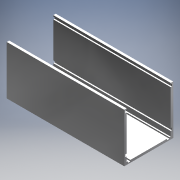
# Autodesk Inventor part: CompactSlidePart1
Saved by Autodesk Inventor 2019 (Build 230136000, 136)
## iProperties
Created: 2017-11-11
Part Number: CompactSlidePart1
Material: Aluminum 6061
Document SubType Name: Modeling
Designer: User
Density: 2.7 g/cm^3
Appearance: Aluminum - Flat
Mass: 1825.11 g
Surface Area: 2444.35 cm^2
Volume: 675.966 cm^3
Author: User
Autodesk Inventor part; units mm, degrees
ref_plane "YZ Plane" through (0, 0, 0) normal (1, 0, 0) x (0, 1, 0)
ref_plane "XZ Plane" through (0, 0, 0) normal (0, 1, 0) x (-1, 0, 0)
ref_plane "XY Plane" through (0, 0, 0) normal (0, 0, 1) x (1, 0, 0)
sketch "Sketch1" plane through (0, 0, 0) normal (1, 0, 0) x (0, 1, 0)
  line L0 (0, 0) -> (-127, 0)
  line L1 (-127, 0) -> (-127, -127)
  line L2 (-127, -127) -> (0, -127)
  line L3 (0, -127) -> (0, -120.65)
  line L4 (0, -6.35) -> (0, 0)
  line L5 (0, -6.35) -> (-3.175, -6.35)
  line L6 (-3.175, -6.35) -> (-3.175, -3.175)
  line L7 (-3.175, -3.175) -> (-9.525, -3.175)
  line L8 (-9.525, -3.175) -> (-9.525, -6.35)
  line L9 (-3.175, -6.35) -> (0, -6.35)
  line L10 (0, -120.65) -> (-3.175, -120.65)
  line L11 (-3.175, -120.65) -> (-3.175, -123.825)
  line L12 (-3.175, -123.825) -> (-9.525, -123.825)
  line L13 (-9.525, -123.825) -> (-9.525, -120.65)
  line L14 (0, -120.65) -> (-3.175, -120.65)
  line L15 (-120.65, -6.35) -> (-120.65, -9.525)
  line L16 (-120.65, -9.525) -> (-123.825, -9.525)
  line L17 (-123.825, -9.525) -> (-123.825, -15.875)
  line L18 (-123.825, -15.875) -> (-120.65, -15.875)
  line L19 (-120.65, -9.525) -> (-120.65, -6.35)
  line L20 (-120.65, -120.65) -> (-120.65, -117.475)
  line L21 (-120.65, -117.475) -> (-123.825, -117.475)
  line L22 (-123.825, -117.475) -> (-123.825, -111.125)
  line L23 (-123.825, -111.125) -> (-120.65, -111.125)
  line L24 (-120.65, -120.65) -> (-120.65, -117.475)
  line L25 (-120.65, -111.125) -> (-120.65, -15.875)
  line L26 (-120.65, -6.35) -> (-107.95, -6.35)
  line L27 (-107.95, -6.35) -> (-107.95, -3.175)
  line L28 (-107.95, -3.175) -> (-101.6, -3.175)
  line L29 (-101.6, -3.175) -> (-101.6, -6.35)
  line L30 (-120.65, -6.35) -> (-107.95, -6.35)
  line L31 (-101.6, -6.35) -> (-9.525, -6.35)
  line L32 (-120.65, -120.65) -> (-107.95, -120.65)
  line L33 (-107.95, -120.65) -> (-107.95, -123.825)
  line L34 (-107.95, -123.825) -> (-101.6, -123.825)
  line L35 (-101.6, -123.825) -> (-101.6, -120.65)
  line L36 (-9.525, -120.65) -> (-101.6, -120.65)
  line L37 (-107.95, -120.65) -> (-120.65, -120.65)
  dimension "d0" = 127
  dimension "d1" = 127
  dimension "d2" = 6.35
  dimension "d3" = 120.65
  dimension "d4" = 114.3
  dimension "d5" = 3.175
  dimension "d9" = 3.175
  dimension "d10" = 3.175
  dimension "d11" = 3.175
  dimension "d12" = 6.35
  dimension "d13" = 3.175
  dimension "d14" = 3.175
  dimension "d15" = 6.35
  dimension "d16" = 3.175
  dimension "d17" = 3.175
  dimension "d18" = 6.35
  dimension "d21" = 12.7
  dimension "d22" = 3.175
  dimension "d23" = 6.35
  dimension "d24" = 12.7
  dimension "d25" = 3.175
  dimension "d26" = 6.35
  constraints: 76 end point, 46 perpendicular, 4 horizontal, 3 parallel
  measures "d0" distance of L0.start L0.end
  measures "d1" distance of L0.end L1.end
  measures "d2" distance of L2.end L3.end
  measures "d3" distance of L3.end L20.start
  measures "d4" distance of L20.start L15.start
  measures "d5" distance of L4.start L5.end
  measures "d9" distance between parallel lines of L5 L7
  measures "d10" distance of L3.end L10.end
  measures "d11" distance of L10.end L11.end
  measures "d12" distance of L11.end L12.end
  measures "d13" distance of L15.start L15.end
  measures "d14" distance of L15.end L16.end
  measures "d15" distance of L16.end L17.end
  measures "d16" distance of L20.start L20.end
  measures "d17" distance of L20.end L21.end
  measures "d18" distance of L21.end L22.end
  measures "d21" distance of L15.start L26.end
  measures "d22" distance of L26.end L27.end
  measures "d23" distance of L27.end L28.end
  measures "d24" distance of L20.start L32.end
  measures "d25" distance of L32.end L33.end
  measures "d26" distance of L33.end L34.end
extrude "Extrusion1" add sketch "Sketch1" along normal blind 304.8
body "Solid1"
